Autodesk Inventor part; units mm, degrees
(part 2 of 2)
  arc A351 (-550.3904, 224.5) -> (-550.3904, 217.8) centre (-550.3904, 221.15) ccw
  line L359 (-387.0904, 237.9) -> (-430.3904, 237.9)
  arc A352 (-430.3904, 237.9) -> (-430.3904, 231.2) centre (-430.3904, 234.55) ccw
  line L360 (-430.3904, 231.2) -> (-387.0904, 231.2)
  arc A353 (-387.0904, 231.2) -> (-387.0904, 237.9) centre (-387.0904, 234.55) ccw
  arc A354 (-447.0904, 231.2) -> (-447.0904, 237.9) centre (-447.0904, 234.55) ccw
  line L361 (-447.0904, 237.9) -> (-490.3904, 237.9)
  line L362 (-490.3904, 231.2) -> (-447.0904, 231.2)
  arc A355 (-490.3904, 237.9) -> (-490.3904, 231.2) centre (-490.3904, 234.55) ccw
  arc A356 (-507.0904, 231.2) -> (-507.0904, 237.9) centre (-507.0904, 234.55) ccw
  line L363 (-507.0904, 237.9) -> (-550.3904, 237.9)
  line L364 (-550.3904, 231.2) -> (-507.0904, 231.2)
  arc A357 (-550.3904, 237.9) -> (-550.3904, 231.2) centre (-550.3904, 234.55) ccw
  line L365 (-387.0904, 251.3) -> (-430.3904, 251.3)
  arc A358 (-430.3904, 251.3) -> (-430.3904, 244.6) centre (-430.3904, 247.95) ccw
  line L366 (-430.3904, 244.6) -> (-387.0904, 244.6)
  arc A359 (-387.0904, 244.6) -> (-387.0904, 251.3) centre (-387.0904, 247.95) ccw
  arc A360 (-447.0904, 244.6) -> (-447.0904, 251.3) centre (-447.0904, 247.95) ccw
  line L367 (-447.0904, 251.3) -> (-490.3904, 251.3)
  line L368 (-490.3904, 244.6) -> (-447.0904, 244.6)
  arc A361 (-490.3904, 251.3) -> (-490.3904, 244.6) centre (-490.3904, 247.95) ccw
  arc A362 (-507.0904, 244.6) -> (-507.0904, 251.3) centre (-507.0904, 247.95) ccw
  line L369 (-507.0904, 251.3) -> (-550.3904, 251.3)
  line L370 (-550.3904, 244.6) -> (-507.0904, 244.6)
  arc A363 (-550.3904, 251.3) -> (-550.3904, 244.6) centre (-550.3904, 247.95) ccw
  line L371 (-387.0904, 264.7) -> (-430.3904, 264.7)
  arc A364 (-430.3904, 264.7) -> (-430.3904, 258) centre (-430.3904, 261.35) ccw
  line L372 (-430.3904, 258) -> (-387.0904, 258)
  arc A365 (-387.0904, 258) -> (-387.0904, 264.7) centre (-387.0904, 261.35) ccw
  arc A366 (-447.0904, 258) -> (-447.0904, 264.7) centre (-447.0904, 261.35) ccw
  line L373 (-447.0904, 264.7) -> (-490.3904, 264.7)
  line L374 (-490.3904, 258) -> (-447.0904, 258)
  arc A367 (-490.3904, 264.7) -> (-490.3904, 258) centre (-490.3904, 261.35) ccw
  arc A368 (-507.0904, 258) -> (-507.0904, 264.7) centre (-507.0904, 261.35) ccw
  line L375 (-507.0904, 264.7) -> (-550.3904, 264.7)
  line L376 (-550.3904, 258) -> (-507.0904, 258)
  arc A369 (-550.3904, 264.7) -> (-550.3904, 258) centre (-550.3904, 261.35) ccw
  line L377 (-387.0904, 278.1) -> (-430.3904, 278.1)
  arc A370 (-430.3904, 278.1) -> (-430.3904, 271.4) centre (-430.3904, 274.75) ccw
  line L378 (-430.3904, 271.4) -> (-387.0904, 271.4)
  arc A371 (-387.0904, 271.4) -> (-387.0904, 278.1) centre (-387.0904, 274.75) ccw
  arc A372 (-447.0904, 271.4) -> (-447.0904, 278.1) centre (-447.0904, 274.75) ccw
  line L379 (-447.0904, 278.1) -> (-490.3904, 278.1)
  line L380 (-490.3904, 271.4) -> (-447.0904, 271.4)
  arc A373 (-490.3904, 278.1) -> (-490.3904, 271.4) centre (-490.3904, 274.75) ccw
  arc A374 (-507.0904, 271.4) -> (-507.0904, 278.1) centre (-507.0904, 274.75) ccw
  line L381 (-507.0904, 278.1) -> (-550.3904, 278.1)
  line L382 (-550.3904, 271.4) -> (-507.0904, 271.4)
  arc A375 (-550.3904, 278.1) -> (-550.3904, 271.4) centre (-550.3904, 274.75) ccw
  line L383 (-387.0904, 291.5) -> (-430.3904, 291.5)
  arc A376 (-430.3904, 291.5) -> (-430.3904, 284.8) centre (-430.3904, 288.15) ccw
  line L384 (-430.3904, 284.8) -> (-387.0904, 284.8)
  arc A377 (-387.0904, 284.8) -> (-387.0904, 291.5) centre (-387.0904, 288.15) ccw
  arc A378 (-447.0904, 284.8) -> (-447.0904, 291.5) centre (-447.0904, 288.15) ccw
  line L385 (-447.0904, 291.5) -> (-490.3904, 291.5)
  line L386 (-490.3904, 284.8) -> (-447.0904, 284.8)
  arc A379 (-490.3904, 291.5) -> (-490.3904, 284.8) centre (-490.3904, 288.15) ccw
  arc A380 (-507.0904, 284.8) -> (-507.0904, 291.5) centre (-507.0904, 288.15) ccw
  line L387 (-507.0904, 291.5) -> (-550.3904, 291.5)
  line L388 (-550.3904, 284.8) -> (-507.0904, 284.8)
  arc A381 (-550.3904, 291.5) -> (-550.3904, 284.8) centre (-550.3904, 288.15) ccw
  line L389 (-387.0904, 304.9) -> (-430.3904, 304.9)
  arc A382 (-430.3904, 304.9) -> (-430.3904, 298.2) centre (-430.3904, 301.55) ccw
  line L390 (-430.3904, 298.2) -> (-387.0904, 298.2)
  arc A383 (-387.0904, 298.2) -> (-387.0904, 304.9) centre (-387.0904, 301.55) ccw
  arc A384 (-447.0904, 298.2) -> (-447.0904, 304.9) centre (-447.0904, 301.55) ccw
  line L391 (-447.0904, 304.9) -> (-490.3904, 304.9)
  line L392 (-490.3904, 298.2) -> (-447.0904, 298.2)
  arc A385 (-490.3904, 304.9) -> (-490.3904, 298.2) centre (-490.3904, 301.55) ccw
  arc A386 (-507.0904, 298.2) -> (-507.0904, 304.9) centre (-507.0904, 301.55) ccw
  line L393 (-507.0904, 304.9) -> (-550.3904, 304.9)
  line L394 (-550.3904, 298.2) -> (-507.0904, 298.2)
  arc A387 (-550.3904, 304.9) -> (-550.3904, 298.2) centre (-550.3904, 301.55) ccw
  line L395 (-387.0904, 318.3) -> (-430.3904, 318.3)
  arc A388 (-430.3904, 318.3) -> (-430.3904, 311.6) centre (-430.3904, 314.95) ccw
  line L396 (-430.3904, 311.6) -> (-387.0904, 311.6)
  arc A389 (-387.0904, 311.6) -> (-387.0904, 318.3) centre (-387.0904, 314.95) ccw
  arc A390 (-447.0904, 311.6) -> (-447.0904, 318.3) centre (-447.0904, 314.95) ccw
  line L397 (-447.0904, 318.3) -> (-490.3904, 318.3)
  line L398 (-490.3904, 311.6) -> (-447.0904, 311.6)
  arc A391 (-490.3904, 318.3) -> (-490.3904, 311.6) centre (-490.3904, 314.95) ccw
  arc A392 (-507.0904, 311.6) -> (-507.0904, 318.3) centre (-507.0904, 314.95) ccw
  line L399 (-507.0904, 318.3) -> (-550.3904, 318.3)
  line L400 (-550.3904, 311.6) -> (-507.0904, 311.6)
  arc A393 (-550.3904, 318.3) -> (-550.3904, 311.6) centre (-550.3904, 314.95) ccw
  line L401 (-387.0904, 331.7) -> (-430.3904, 331.7)
  arc A394 (-430.3904, 331.7) -> (-430.3904, 325) centre (-430.3904, 328.35) ccw
  line L402 (-430.3904, 325) -> (-387.0904, 325)
  arc A395 (-387.0904, 325) -> (-387.0904, 331.7) centre (-387.0904, 328.35) ccw
  arc A396 (-447.0904, 325) -> (-447.0904, 331.7) centre (-447.0904, 328.35) ccw
  line L403 (-447.0904, 331.7) -> (-490.3904, 331.7)
  line L404 (-490.3904, 325) -> (-447.0904, 325)
  arc A397 (-490.3904, 331.7) -> (-490.3904, 325) centre (-490.3904, 328.35) ccw
  arc A398 (-507.0904, 325) -> (-507.0904, 331.7) centre (-507.0904, 328.35) ccw
  line L405 (-507.0904, 331.7) -> (-550.3904, 331.7)
  line L406 (-550.3904, 325) -> (-507.0904, 325)
  arc A399 (-550.3904, 331.7) -> (-550.3904, 325) centre (-550.3904, 328.35) ccw
  line L407 (-387.0904, 345.1) -> (-430.3904, 345.1)
  arc A400 (-430.3904, 345.1) -> (-430.3904, 338.4) centre (-430.3904, 341.75) ccw
  line L408 (-430.3904, 338.4) -> (-387.0904, 338.4)
  arc A401 (-387.0904, 338.4) -> (-387.0904, 345.1) centre (-387.0904, 341.75) ccw
  arc A402 (-447.0904, 338.4) -> (-447.0904, 345.1) centre (-447.0904, 341.75) ccw
  line L409 (-447.0904, 345.1) -> (-490.3904, 345.1)
  line L410 (-490.3904, 338.4) -> (-447.0904, 338.4)
  arc A403 (-490.3904, 345.1) -> (-490.3904, 338.4) centre (-490.3904, 341.75) ccw
  arc A404 (-507.0904, 338.4) -> (-507.0904, 345.1) centre (-507.0904, 341.75) ccw
  line L411 (-507.0904, 345.1) -> (-550.3904, 345.1)
  line L412 (-550.3904, 338.4) -> (-507.0904, 338.4)
  arc A405 (-550.3904, 345.1) -> (-550.3904, 338.4) centre (-550.3904, 341.75) ccw
  line L413 (-387.0904, 358.5) -> (-430.3904, 358.5)
  arc A406 (-430.3904, 358.5) -> (-430.3904, 351.8) centre (-430.3904, 355.15) ccw
  line L414 (-430.3904, 351.8) -> (-387.0904, 351.8)
  arc A407 (-387.0904, 351.8) -> (-387.0904, 358.5) centre (-387.0904, 355.15) ccw
  arc A408 (-447.0904, 351.8) -> (-447.0904, 358.5) centre (-447.0904, 355.15) ccw
  line L415 (-447.0904, 358.5) -> (-490.3904, 358.5)
  line L416 (-490.3904, 351.8) -> (-447.0904, 351.8)
  arc A409 (-490.3904, 358.5) -> (-490.3904, 351.8) centre (-490.3904, 355.15) ccw
  arc A410 (-507.0904, 351.8) -> (-507.0904, 358.5) centre (-507.0904, 355.15) ccw
  line L417 (-507.0904, 358.5) -> (-550.3904, 358.5)
  line L418 (-550.3904, 351.8) -> (-507.0904, 351.8)
  arc A411 (-550.3904, 358.5) -> (-550.3904, 351.8) centre (-550.3904, 355.15) ccw
  point P0 (-288.7396, 20.15)
  point P1 (-348.7404, 20.15)
  dimension "d13" = 50
  dimension "d22" = 60
  dimension "d31" = 13.4
  dimension "d38" = 13.4
  constraints: 834 end point, 828 point on circle, 621 symmetric about line, 412 centre point, 4 point on line, 4 tangent, 3 midpoint, 2 vertical, 1 horizontal, 1 parallel, 1226 other
  measures "d13" distance of L5.start L5.end
  measures "d22" distance of L6.start L8.start
  measures "d31" distance of L7.start L14.start
  measures "d38" distance of L8.start L62.start
extrude "Extrusión7" cut sketch "Boceto6" against normal blind 10 contours L6 A1 L7 A0 | L8 A3 L9 A2 | L10 A5 L11 A4 | L12 A7 L13 A6 | L14 A9 L15 A8 | L16 A11 L17 A10 | L18 A13 L19 A12 | L20 A15 L21 A14 | L22 A17 L23 A16 | L24 A19 L25 A18 | L26 A21 L27 A20 | L28 A23 L29 A22 | L30 A25 L31 A24 | L32 A27 L33 A26 | L34 A29 L35 A28 | L36 A31 L37 A30 | L38 A33 L39 A32 | L40 A35 L41 A34 | L42 A37 L43 A36 | L44 A39 L45 A38 | L46 A41 L47 A40 | L48 A43 L49 A42 | L50 A45 L51 A44 | L52 A47 L53 A46 | L54 A49 L55 A48 | L56 A51 L57 A50 | L58 A53 L59 A52 | L60 A55 L61 A54 | L62 A56 L63 A57 | L64 A59 L65 A58 | L66 A61 L67 A60 | L68 A62 L69 A63 | L70 A65 L71 A64 | L72 A67 L73 A66 | L74 A68 L75 A69 | L76 A71 L77 A70 | L78 A73 L79 A72 | L80 A74 L81 A75 | L82 A77 L83 A76 | L84 A79 L85 A78 | L86 A80 L87 A81 | L88 A83 L89 A82 | L90 A85 L91 A84 | L92 A86 L93 A87 | L94 A89 L95 A88 | L96 A91 L97 A90 | L98 A92 L99 A93 | L100 A95 L101 A94 | L102 A97 L103 A96 | L104 A98 L105 A99 | L106 A101 L107 A100 | L108 A103 L109 A102 | L110 A104 L111 A105 | L112 A107 L113 A106 | L114 A109 L115 A108 | L116 A110 L117 A111 | L118 A113 L119 A112 | L120 A115 L121 A114 | L122 A116 L123 A117 | L124 A119 L125 A118 | L126 A121 L127 A120 | L128 A122 L129 A123 | L130 A125 L131 A124 | L132 A127 L133 A126 | L134 A128 L135 A129 | L136 A131 L137 A130 | L138 A133 L139 A132 | L140 A134 L141 A135 | L142 A137 L143 A136 | L144 A139 L145 A138 | L146 A140 L147 A141 | L148 A143 L149 A142 | L150 A145 L151 A144 | L152 A146 L153 A147 | L154 A149 L155 A148 | L156 A151 L157 A150 | L158 A152 L159 A153 | L160 A155 L161 A154 | L162 A157 L163 A156 | L164 A158 L165 A159 | L166 A161 L167 A160 | L168 A163 L169 A162 | L170 A164 L171 A165 | L172 A167 L173 A166 | L174 A169 L175 A168 | L176 A170 L177 A171 | L178 A173 L179 A172 | L180 A175 L181 A174 | L182 A176 L183 A177 | L184 A179 L185 A178 | L186 A181 L187 A180 | L188 A182 L189 A183 | L190 A185 L191 A184 | L192 A187 L193 A186 | L194 A188 L195 A189 | L196 A191 L197 A190 | L198 A193 L199 A192 | L200 A194 L201 A195 | L202 A197 L203 A196 | L204 A199 L205 A198 | L206 A200 L207 A201 | L208 A203 L209 A202 | L210 A205 L211 A204 | A206 L214 A207 L213 | A208 L216 A209 L215 | A210 L218 A211 L217 | A212 L220 A213 L219 | A214 L222 A215 L221 | A216 L224 A217 L223 | A218 L226 A219 L225 | A220 L228 A221 L227 | A222 L230 A223 L229 | A224 L232 A225 L231 | A226 L234 A227 L233 | A228 L236 A229 L235 | A230 L238 A231 L237 | A232 L240 A233 L239 | A234 L242 A235 L241 | A236 L244 A237 L243 | A238 L246 A239 L245 | A240 L248 A241 L247 | A242 L250 A243 L249 | A244 L252 A245 L251 | A246 L254 A247 L253 | A248 L256 A249 L255 | A250 L258 A251 L257 | A252 L260 A253 L259 | A254 L262 A255 L261 | A256 L264 A257 L263 | A258 L266 A259 L265 | A260 L268 A261 L267 | A263 L270 A262 L269 | L272 A265 L271 A264 | L274 A267 L273 A266 | A269 L276 A268 L275 | L278 A271 L277 A270 | L280 A273 L279 A272 | A275 L282 A274 L281 | L284 A277 L283 A276 | L286 A279 L285 A278 | A281 L288 A280 L287 | L290 A283 L289 A282 | L292 A285 L291 A284 | A287 L294 A286 L293 | L296 A289 L295 A288 | L298 A291 L297 A290 | A293 L300 A292 L299 | L302 A295 L301 A294 | L304 A297 L303 A296 | A299 L306 A298 L305 | L308 A301 L307 A300 | L310 A303 L309 A302 | A305 L312 A304 L311 | L314 A307 L313 A306 | L316 A309 L315 A308 | A311 L318 A310 L317 | L320 A313 L319 A312 | L322 A315 L321 A314 | A317 L324 A316 L323 | L326 A319 L325 A318 | L328 A321 L327 A320 | A323 L330 A322 L329 | L332 A325 L331 A324 | L334 A327 L333 A326 | A329 L336 A328 L335 | L338 A331 L337 A330 | L340 A333 L339 A332 | A335 L342 A334 L341 | L344 A337 L343 A336 | L346 A339 L345 A338 | A341 L348 A340 L347 | L350 A343 L349 A342 | L352 A345 L351 A344 | A347 L354 A346 L353 | L356 A349 L355 A348 | L358 A351 L357 A350 | A353 L360 A352 L359 | L362 A355 L361 A354 | L364 A357 L363 A356 | A359 L366 A358 L365 | L368 A361 L367 A360 | L370 A363 L369 A362 | A365 L372 A364 L371 | L374 A367 L373 A366 | L376 A369 L375 A368 | A371 L378 A370 L377 | L380 A373 L379 A372 | L382 A375 L381 A374 | A377 L384 A376 L383 | L386 A379 L385 A378 | L388 A381 L387 A380 | A383 L390 A382 L389 | L392 A385 L391 A384 | L394 A387 L393 A386 | A389 L396 A388 L395 | L398 A391 L397 A390 | L400 A393 L399 A392 | A395 L402 A394 L401 | L404 A397 L403 A396 | L406 A399 L405 A398 | A401 L408 A400 L407 | L410 A403 L409 A402 | L412 A405 L411 A404 | A407 L414 A406 L413 | L416 A409 L415 A408 | L418 A411 L417 A410
sketch "Boceto7" plane through (-637.48, 0.76, 0) normal (0, 0, 1) x (1, 0, 0)
  circle A0 centre (76.24, -127.61) radius 3.175
  circle A1 centre (561.24, -127.61) radius 3.175
  point P0 (637.48, -0.76)
  dimension "d45" = 6.35
  dimension "d46" = 6.35
  constraints: 2 centre point
  measures "d45" diameter of A0
  measures "d46" diameter of A1
extrude "Extrusión8" cut sketch "Boceto7" against normal up to surface (0.76 mm away)
